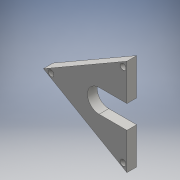
# Autodesk Inventor part: Support extruder v1
Saved by Autodesk Inventor 2016 (Build 200138000, 138)
## iProperties
Created: 2016-07-05
Part Number: Support extruder v1
Material: Generic
Document SubType Name: Modeling
Designer: Thetheos
Density: 1 g/cm^3
Appearance: Default
Author: Thetheos
Autodesk Inventor part; units mm, degrees
ref_plane "YZ Plane" through (0, 0, 0) normal (1, 0, 0) x (0, 1, 0)
ref_plane "XZ Plane" through (0, 0, 0) normal (0, 1, 0) x (-1, 0, 0)
ref_plane "XY Plane" through (0, 0, 0) normal (0, 0, 1) x (1, 0, 0)
sketch "Sketch1" plane through (0, 0, 0) normal (0, 1, 0) x (-1, 0, 0)
  circle A0 centre (0, 0) radius 1.5
  circle A1 centre (0, -43) radius 1.5
  circle A2 centre (37.2391, -21.5) radius 1.5
  line L0 (12.413, -15.5) -> (0, -15.5)
  line L1 (12.413, -27.5) -> (0, -27.5)
  arc A3 (12.413, -27.5) -> (12.413, -15.5) centre (12.413, -21.5) ccw
  line L2 (-2, 3.4641) -> (41.2391, -21.5)
  line L3 (41.2391, -21.5) -> (-2, -46.4641)
  line L4 (0, -15.5) -> (-2, -15.5)
  line L5 (0, -27.5) -> (-2, -27.5)
  line L6 (-2, -27.5) -> (-2, -46.4641)
  line L7 (-2, 3.4641) -> (-2, -15.5)
  dimension "d0" = 3
  dimension "d1" = 3
  dimension "d2" = 43
  dimension "d4" = 3
  constraints: 16 end point, 4 centre point, 2 coincident, 2 point on circle, 2 tangent, 1 perpendicular, 5 other
  measures "d0" diameter of A0
  measures "d1" diameter of A1
  measures "d2" distance of point (0, 0) A1.centre
  measures "d4" diameter of A2
extrude "Extrusion1" add sketch "Sketch1" along normal blind 5
body "Solid1"
